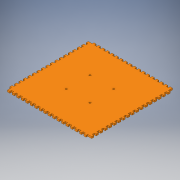
# Autodesk Inventor part: 000.201 - Дно
Saved by Autodesk Inventor 2019 (Build 230136000, 136)
## iProperties
Created: 2020-02-27
Part Number: 000.201 - Дно
Material: Типовые
Document SubType Name: Modeling
Designer: Петров Иван
Density: 1 g/cm^3
Appearance: Оранжевый
Author: Петров Иван
Autodesk Inventor part; units mm, degrees
ref_plane "YZ Plane" through (0, 0, 0) normal (1, 0, 0) x (0, 1, 0)
ref_plane "XZ Plane" through (0, 0, 0) normal (0, 1, 0) x (-1, 0, 0)
ref_plane "XY Plane" through (0, 0, 0) normal (0, 0, 1) x (1, 0, 0)
sketch "Эскиз1" plane through (0, 0, 0) normal (0, 1, 0) x (-1, 0, 0)
  line L0 (-72, 72) -> (72, 72)
  line L1 (72, 72) -> (72, -72)
  line L2 (72, -72) -> (-72, -72)
  line L3 (-72, -72) -> (-72, 72)
  line L4 (-72, 72) -> (72, -72) construction
  line L5 (72, 72) -> (-72, -72) construction
  point P0 (0, 0)
  dimension "d0" = 144
  dimension "d1" = 144
  constraints: 12 end point, 2 midpoint, 2 parallel, 1 horizontal, 1 perpendicular
  measures "d0" distance of L1.end L2.end
  measures "d1" distance of L0.end L1.end
extrude "Выдавливание1" add sketch "Эскиз1" along normal blind 3
sketch "Эскиз2" plane through (0, 3, 0) normal (0, 1, 0) x (1, 0, 0)
  line L0 (-72, 72) -> (-72, -72) projected
  line L1 (-72, -72) -> (-68, -72)
  line L2 (-68, -72) -> (-68, -75)
  line L3 (-68, -75) -> (-72, -75)
  line L4 (-72, -75) -> (-72, -72)
  point P0 (0, 0)
  dimension "d4" = 4
  dimension "d5" = 3
  constraints: 8 end point, 2 parallel, 1 horizontal, 1 perpendicular
  measures "d4" distance of L2.end L3.end
  measures "d5" distance of L1.end L2.end
extrude "Выдавливание2" add sketch "Эскиз2" against normal blind 3
pattern_linear "Прямоуг.массив1" count 18 spacing 8 along (1, 0, 0) of "Выдавливание2"
pattern_circular "Круговой массив1" count 4 over 360 about axis through (0, -10, 0) along (0, 1, 0) of "Выдавливание2", "Прямоуг.массив1"
sketch "Эскиз3" plane through (0, 3, 0) normal (0, 1, 0) x (1, 0, 0)
  line L0 (-37.7, 64.1456) -> (-37.7, 60.8956)
  line L1 (-37.7, 60.8956) -> (-30.7, 60.8956)
  line L2 (-30.7, 60.8956) -> (-30.7, 70.3956)
  line L3 (-30.7, 70.3956) -> (-36.7, 70.3956)
  arc A0 (-36.7, 70.3956) -> (-37.7, 69.3956) centre (-36.7, 69.3956) ccw
  line L4 (-37.7, 69.3956) -> (-37.7, 66.5456)
  line L5 (-37.7, 66.5456) -> (-36.634, 66.5456)
  arc A1 (-36.634, 64.1456) -> (-36.634, 66.5456) centre (-34.85, 65.3456) ccw
  line L6 (-36.634, 64.1456) -> (-37.7, 64.1456)
  line L7 (-37.7, 59.8956) -> (-30.7, 59.8956)
  line L8 (-37.7, 59.8956) -> (-37.7, 56.6456)
  line L9 (-37.7, 56.6456) -> (-36.634, 56.6456)
  arc A2 (-36.634, 54.2456) -> (-36.634, 56.6456) centre (-34.85, 55.4456) ccw
  line L10 (-36.634, 54.2456) -> (-37.7, 54.2456)
  line L11 (-37.7, 54.2456) -> (-37.7, 51.3956)
  arc A3 (-37.7, 51.3956) -> (-36.7, 50.3956) centre (-36.7, 51.3956) ccw
  line L12 (-36.7, 50.3956) -> (-30.7, 50.3956)
  line L13 (-30.7, 50.3956) -> (-30.7, 59.8956)
  line L14 (-37.7, 60.8956) -> (-37.7, 59.8956)
  line L15 (17, 60.8956) -> (17, 59.8956)
  line L16 (10, 59.8956) -> (17, 59.8956)
  line L17 (10, 50.3956) -> (10, 59.8956)
  line L18 (16, 50.3956) -> (10, 50.3956)
  arc A4 (16, 50.3956) -> (17, 51.3956) centre (16, 51.3956) ccw
  line L19 (17, 54.2456) -> (17, 51.3956)
  line L20 (15.934, 54.2456) -> (17, 54.2456)
  arc A5 (15.934, 56.6456) -> (15.934, 54.2456) centre (14.15, 55.4456) ccw
  line L21 (17, 56.6456) -> (15.934, 56.6456)
  line L22 (17, 59.8956) -> (17, 56.6456)
  line L23 (10, 60.8956) -> (10, 70.3956)
  line L24 (10, 60.8956) -> (17, 60.8956)
  line L25 (17, 64.1456) -> (17, 60.8956)
  line L26 (15.934, 64.1456) -> (17, 64.1456)
  arc A6 (15.934, 66.5456) -> (15.934, 64.1456) centre (14.15, 65.3456) ccw
  line L27 (17, 66.5456) -> (15.934, 66.5456)
  line L28 (17, 69.3956) -> (17, 66.5456)
  arc A7 (17, 69.3956) -> (16, 70.3956) centre (16, 69.3956) ccw
  line L29 (10, 70.3956) -> (16, 70.3956)
  line L30 (0, 70.3956) -> (10, 70.3956)
  line L31 (-30.7, 70.3956) -> (0, 70.3956)
  line L32 (-30.7, 50.3956) -> (0, 50.3956)
  line L33 (0, 50.3956) -> (10, 50.3956)
  circle A8 centre (0, 60.3956) radius 5.4
  circle A9 centre (0, 60.3956) radius 6.5
  circle A10 centre (0, 60.3956) radius 1.25
  circle A11 centre (-34.85, 55.4456) radius 2.15
  circle A12 centre (-34.85, 65.3456) radius 2.15
  circle A13 centre (14.15, 65.3456) radius 2.15
  circle A14 centre (14.15, 55.4456) radius 2.15
  line L34 (15.934, 54.2456) -> (17, 54.2456)
  line L35 (17, 56.6456) -> (15.934, 56.6456)
  line L36 (17, 54.2456) -> (17, 56.6456)
  line L37 (17, 56.6456) -> (17, 66.5456)
  line L38 (17, 66.5456) -> (15.934, 66.5456)
  line L39 (17, 64.1456) -> (17, 66.5456)
  line L40 (-37.7, 64.1456) -> (-37.7, 56.6456)
  line L41 (-37.7, 66.5456) -> (-37.7, 64.1456)
  line L42 (-37.7, 56.6456) -> (-36.634, 56.6456)
  line L43 (-37.7, 56.6456) -> (-37.7, 54.2456)
  point P0 (0, 0)
  point P1 (-10.35, 50.3956)
  constraints: 88 end point, 16 point on circle, 15 centre point, 4 coincident, 3 concentric, 3 vertical, 1 collinear, 1 perpendicular
extrude "Выдавливание3" [suppressed]
sketch "Эскиз4" plane through (0, 3, 0) normal (0, 1, 0) x (1, 0, 0)
  arc A0 (-18, 26.5) -> (-26.5, 18) centre (-18, 18) ccw
  line L0 (-26.5, -18) -> (-26.5, 18)
  arc A1 (-26.5, -18) -> (-18, -26.5) centre (-18, -18) ccw
  line L1 (18, -26.5) -> (-18, -26.5)
  arc A2 (18, -26.5) -> (26.5, -18) centre (18, -18) ccw
  line L2 (26.5, 18) -> (26.5, -18)
  arc A3 (26.5, 18) -> (18, 26.5) centre (18, 18) ccw
  line L3 (-18, 26.5) -> (18, 26.5)
  circle A4 centre (-21.2132, 21.2132) radius 1.5
  circle A5 centre (-21.2132, -21.2132) radius 1.5
  circle A6 centre (21.2132, -21.2132) radius 1.5
  circle A7 centre (21.2132, 21.2132) radius 1.5
  line L4 (18, 18) -> (-18, 18)
  line L5 (-18, 18) -> (-18, -18)
  line L6 (-18, -18) -> (18, -18)
  line L7 (18, -18) -> (18, 18)
  point P0 (0, 0)
  point P1 (0, 0)
  point P2 (0, 0)
  constraints: 16 end point, 8 centre point, 8 point on circle, 2 parallel, 1 horizontal, 1 perpendicular
extrude "Выдавливание4" cut sketch "Эскиз4" against normal blind 10 contours A4 | A5 | A6 | A7
